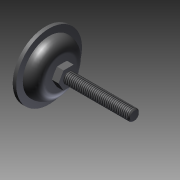
# Autodesk Inventor part: NFJN5-30pad
Saved by Autodesk Inventor 2011 SP1 (Build 150282100, 282)
## iProperties
Created: 2018-01-07
Part Number: NFJN5-30pad
Catalog Web Link: www.cadenas.de
Description: NFJN, NFJNS, NFJNFpad-Adjustment Pads - Standard
Vendor: MISUMI
Document SubType Name: Modeling
Designer: psAdmin
Manufacturer: MISUMI
Mass: 3.98005 g
Surface Area: 24.2312 cm^2
Volume: 3.98005 cm^3
Density: 1 g/cm^3
Category: PARTsolutions
Company: MISUMI
Title: NFJN5-30pad
Author: Cadenas PARTsolutions
Comments: Adjustment Pads - Standard
PSOL_IDENT_0: {$CADENAS_DATA\23d-libs\misumi\metric\42_casters_leveling_pads\nfjn_pad.prj},202 {VTYP=3D},{NB=NFJN5
PSOL_IDENT_1: -30pad},{LINA=NFJN5-30pad},{NN=NFJN, NFJNS, NFJNFpad},{DATE=24.04.2017 08:10:58},{GEOMDATE=25.07.201
PSOL_IDENT_2: 3 00:00:00},{VERSION=},{LINEID=10},{LINESUBID=-1},{WBVAR=TS,MAT,A,ALT1,ALT2,ALT3}  {NB=NFJN5-30pad},
PSOL_IDENT_3: {LINA=NFJN5-30pad},{KT=DUMMY},{PN=NFJN5-30},{TS=1},{TYPE=NFJN},{MAT=1},{ST=Trivalent Chromate},{M=5}
PSOL_IDENT_4: ,{A=30},{L=40.5},{D=30},{LL1=3.5},{LL2=4.0},{E=5.4},{B=8},{TT=1.6},{AL=1.5},{MASS=15},{ALT1=},{ALT1A=''
PSOL_IDENT_5: ,'Not applicable'},{ALT2=},{ALT2A='','Not applicable'},{ALT3=},{ALT3A='','Not applicable'},{WC=0},{L
PSOL_IDENT_6: WC=0.0},{WK=0},{LWK=0},{W=0},{SC=0},{LSC=0},{WN=0},{LWN=0},{TSA= '1' , 'A Dimension Selectable'  },{
PSOL_IDENT_7: MATA= '1', '1018 Steel Equivalent', '2', '304 Stainless Steel' },{AALG=30,60},{AALGA=30,60},{AALG2=0
PSOL_IDENT_8: },{LA1=40.5},{LA2=65.0},{ALA1=1.5},{MASS1=15}
NN: NFJN, NFJNS, NFJNFpad
NT: Adjustment Pads - Standard
NB: NFJN5-30pad
NBSYN: $PN.pad
LINA: NFJN5-30pad
PN: NFJN5-30
TS: A Dimension Selectable
MAT: 1018 Steel Equivalent
ST: Trivalent Chromate
M: 5
A: 30
L: 40.5
D: 30
LL1: 3.5
LL2: 4.0
E: 5.4
B: 8
TT: 1.6
AL: 1.5
MASS: 15
ALT1: Not applicable
ALT2: Not applicable
ALT3: Not applicable
WC: 0
LWC: 0.0
WK: 0
LWK: 0
W: 0
SC: 0
LSC: 0
WN: 0
LWN: 0
SUPPLIER: MISUMI
ARTICLENO: NFJN5-30pad
BOMINFO: NFJN5-30pad
CREATOR: CADENAS GmbH
Autodesk Inventor part; units mm, degrees
sketch "Sketch_1" plane through (0, 0, 0) normal (0, 0, 1) x (1, 0, 0)
  line L0 (0, 0) -> (40.5, 0)
  line L1 (40.5, 0) -> (40.5, -2.0095)
  line L2 (40.5, -2.0095) -> (40.0095, -2.5)
  line L3 (40.0095, -2.5) -> (10.5, -2.5)
  line L4 (10.5, -2.5) -> (10.5, -5)
  line L5 (10.5, -5) -> (7.6154, -5)
  line L6 (7.6154, -5) -> (7, -2.5)
  line L7 (7, -2.5) -> (7, -7)
  arc A0 (2, -12) -> (7, -7) centre (2, -7) ccw
  line L8 (2, -12) -> (1.6, -12)
  line L9 (1.6, -12) -> (1.6, -15)
  line L10 (1.6, -15) -> (0, -15)
  line L11 (0, -15) -> (0, 0)
  line L12 (0, 0) -> (40.5, 0)
  constraints: 26 end point, 2 point on circle, 1 centre point
revolve "Revolution1" add sketch "Sketch_1" angle 360 about axis through (0, 0, 0) along (-1, 0, 0)
thread "Thread1" size "M5x0.8" class "6g" standard "ISO Metric profile" full length
sketch "Sketch_2" plane through (10.5, 0, 0) normal (1, 0, 0) x (0, 0, -1)
  circle A0 centre (0, 0) radius 5.2
  line L0 (-4, -2.3094) -> (0, -4.6188)
  line L1 (0, -4.6188) -> (4, -2.3094)
  line L2 (4, -2.3094) -> (4, 2.3094)
  line L3 (4, 2.3094) -> (0, 4.6188)
  line L4 (0, 4.6188) -> (-4, 2.3094)
  line L5 (-4, 2.3094) -> (-4, -2.3094)
  constraints: 12 end point, 1 centre point
extrude "Extrusion1" cut sketch "Sketch_2" against normal blind 3.5
ref_plane "pad_to_dummy_XY" through (0, 0, 0) normal (1, 0, 0) x (0, 0, -1)
ref_plane "pad_to_dummy_YZ" through (0, 0, 0) normal (0, 0, -1) x (0, 1, 0)
ref_plane "pad_to_dummy_ZX" through (0, 0, 0) normal (0, 1, 0) x (1, 0, 0)
ref_plane "pad_to_nut_XY" through (20.25, 0, 0) normal (1, 0, 0) x (0, 0, -1)
ref_plane "pad_to_nut_YZ" through (20.25, 0, 0) normal (0, 0, -1) x (0, 1, 0)
ref_plane "pad_to_nut_ZX" through (20.25, 0, 0) normal (0, 1, 0) x (1, 0, 0)
ref_plane "pad_to_plate_XY" through (36.25, 0, 0) normal (1, 0, 0) x (0, 0, -1)
ref_plane "pad_to_plate_YZ" through (36.25, 0, 0) normal (0, 0, -1) x (0, 1, 0)
ref_plane "pad_to_plate_ZX" through (36.25, 0, 0) normal (0, 1, 0) x (1, 0, 0)
body "Solid1"
